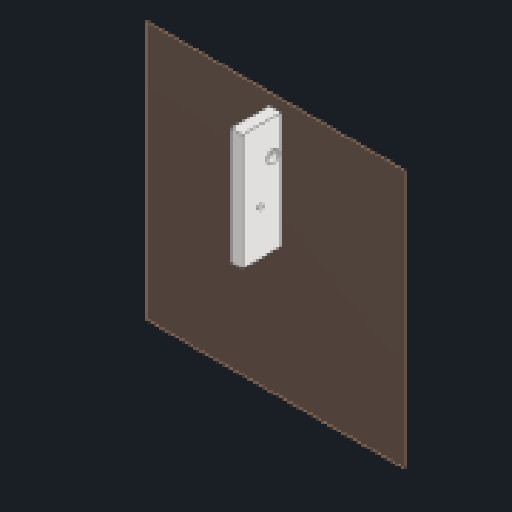
# Autodesk Inventor part: middle_gaer_holder
Saved by Autodesk Inventor 2023 (Build 270158000, 158)
## iProperties
Created: 2024-04-14
Part Number: middle_gaer_holder
Material: Generic
Document SubType Name: Modeling
Designer: szymo
Density: 1 g/cm^3
Appearance: Default
Author: szymo
Autodesk Inventor part; units mm, degrees
ref_plane "YZ Plane" through (0, 0, 0) normal (1, 0, 0) x (0, 1, 0)
ref_plane "XZ Plane" through (0, 0, 0) normal (0, 1, 0) x (-1, 0, 0)
ref_plane "XY Plane" through (0, 0, 0) normal (0, 0, 1) x (1, 0, 0)
ref_plane "Work Plane1" through (0, 0, 0) normal (0, 0, 1) x (1, 0, 0)
sketch "Sketch1" plane through (0, 0, 0) normal (0, 0, 1) x (1, 0, 0)
  line L0 (-74, -73.5) -> (-74, -89.5) projected
  line L1 (-74, -89.5) -> (74, -89.5) projected
  line L2 (74, -89.5) -> (74, -73.5) projected
  line L3 (74, -73.5) -> (89, -73.5) projected
  line L4 (89, -73.5) -> (89, 37.5) projected
  line L5 (89, 37.5) -> (22.5, 37.5) projected
  line L6 (22.5, 37.5) -> (22.5, 89.5) projected
  line L7 (22.5, 89.5) -> (16.5, 89.5) projected
  line L8 (16.5, 89.5) -> (16.5, 37.5) projected
  line L9 (16.5, 37.5) -> (4.5, 37.5) projected
  line L10 (4.5, 37.5) -> (4.5, 89.5) projected
  line L11 (4.5, 89.5) -> (-4.5, 89.5) projected
  line L12 (-4.5, 89.5) -> (-4.5, 37.5) projected
  line L13 (-4.5, 37.5) -> (-16.5, 37.5) projected
  line L14 (-16.5, 37.5) -> (-16.5, 89.5) projected
  line L15 (-16.5, 89.5) -> (-22.5, 89.5) projected
  line L16 (-22.5, 89.5) -> (-22.5, 37.5) projected
  line L17 (-22.5, 37.5) -> (-89, 37.5) projected
  line L18 (-89, 37.5) -> (-89, -73.5) projected
  line L19 (-89, -73.5) -> (-74, -73.5) projected
  circle A0 centre (-29.2, 3.1615) radius 1.8 projected
  line L20 (-22.5, 13.4539) -> (-22.5, 0.9615) projected
  line L21 (-27.2, 13.4539) -> (-22.5, 13.4539) projected
  line L22 (-27.2, 13.4539) -> (-27.2, 5.7703) projected
  line L23 (-27.2, 5.7703) -> (-32.2, 5.7703) projected
  line L24 (-32.2, 0.9615) -> (-32.2, 5.7703) projected
  line L25 (-32.2, 0.9615) -> (-22.5, 0.9615) projected
  circle A1 centre (29.2, 3.1615) radius 1.8 projected
  line L26 (22.5, 13.4539) -> (22.5, 0.9615) projected
  line L27 (32.2, 0.9615) -> (22.5, 0.9615) projected
  line L28 (32.2, 0.9615) -> (32.2, 5.7703) projected
  line L29 (27.2, 5.7703) -> (32.2, 5.7703) projected
  line L30 (27.2, 13.4539) -> (27.2, 5.7703) projected
  line L31 (27.2, 13.4539) -> (22.5, 13.4539) projected
  line L32 (-4.5, 89.5) -> (4.5, 89.5)
  line L33 (4.5, 89.5) -> (4.5, 0.9615)
  line L34 (4.5, 0.9615) -> (-4.5, 0.9615)
  line L35 (-4.5, 0.9615) -> (-4.5, 89.5)
  point P0 (0, 0)
  constraints: 8 end point, 2 collinear, 2 parallel, 1 horizontal, 1 perpendicular
ref_plane "Work Plane2" through (-88.5, 89.5, 29.5) normal (0, 0, 1) x (1, 0, 0)
extrude "Extrusion1" add sketch "Sketch1" along normal up to surface (29.5 mm away) contours L12 L11 L10 L33 L34 L35
sketch "Sketch2" plane through (4.5, 0.9615, 0) normal (1, 0, 0) x (0, 0, -1)
  circle A0 centre (-16.1803, 34.1432) radius 2 projected
  point P0 (0, -0.9615)
extrude "Extrusion2" cut sketch "Sketch2" against normal up to next
sketch "Sketch3" plane through (4.5, 0.9615, 0) normal (1, 0, 0) x (0, 0, -1)
  circle A0 centre (-6.5, 62.5385) radius 5.5 projected
  circle A1 centre (-6.5, 62.5385) radius 4.5
  circle A2 centre (-6.5, 62.5385) radius 4.65
  point P0 (0, -0.9615)
  dimension "d4" = 9
  dimension "d5" = 0.15
  constraints: 2 centre point, 1 coincident
  measures "d4" diameter of A1
  measures "d5" radial gap between concentric circles of A1 A2
extrude "Extrusion3" cut sketch "Sketch3" against normal blind 4.3 contours A1 | A2
sketch "Sketch4" plane through (-4.5, 0.9615, 0) normal (-1, 0, 0) x (0, 0, 1)
  circle A0 centre (6.5, 62.5385) radius 1.2295 projected
  circle A1 centre (6.5, 62.5385) radius 4.65 projected
  circle A2 centre (6.5, 62.5385) radius 4.575
  point P0 (0, -0.9615)
  dimension "d8" = 9.15
  constraints: 1 centre point, 1 coincident
  measures "d8" diameter of A2
extrude "Extrusion4" cut sketch "Sketch4" against normal blind 4.3 contours A0 | A2
sketch "Sketch6" plane through (-4.5, 0.9615, 0) normal (-1, 0, 0) x (0, 0, 1)
  circle A0 centre (5, 20) radius 1.8 projected
  circle A1 centre (23.5, 78.5385) radius 1.8 projected
  point P0 (0, -0.9615)
extrude "Extrusion5" cut sketch "Sketch6" against normal up to surface (9 mm away)
body "Solid1"
